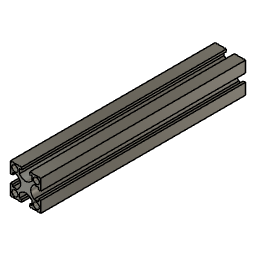
프로파일-135mm (Autodesk Fusion 360 design; units mm, degrees)
Autodesk Fusion 360 part; units mm, degrees
sketch "스케치1" plane through (0, 0, 0) normal (0, 1, 0) x (1, 0, 0)
  line L0 (10, -10) -> (-10, -10)
  line L1 (-10, -10) -> (-10, 10)
  line L2 (-10, 10) -> (10, 10)
  line L3 (10, 10) -> (10, -10)
  line L4 (10, -10) -> (-10, 10) construction
  line L5 (-10, -10) -> (10, 10) construction
  line L6 (10, 0) -> (10, -4.15)
  line L7 (3.3, 0) -> (3.3, 4.15)
  line L8 (3.3, 4.15) -> (10, 4.15)
  line L9 (10, 4.15) -> (10, -4.15)
  line L10 (10, -4.15) -> (3.3, -4.15)
  line L11 (3.3, -4.15) -> (3.3, 4.15)
  line L12 (10, -4.15) -> (8.5, -4.15)
  line L13 (8.5, -4.15) -> (8.5, -2.65)
  line L14 (8.5, -2.65) -> (10, -2.65)
  line L15 (10, -2.65) -> (10, -4.15)
  line L16 (10, 4.15) -> (8.5, 4.15)
  line L17 (8.5, 4.15) -> (8.5, 2.65)
  line L18 (8.5, 2.65) -> (10, 2.65)
  line L19 (10, 2.65) -> (10, 4.15)
  line L20 (8.5, 4.15) -> (5.5, 4.15)
  line L21 (5.5, 4.15) -> (5.5, -4.15)
  line L22 (5.5, -4.15) -> (8.5, -4.15)
  line L23 (8.5, -4.15) -> (8.5, 4.15)
  spline S0 degree 5 poles (5.5, -4.15) (5.3331, -3.984) (5.014, -3.652) (4.579, -3.154) (4.0878, -2.49) (3.6321, -1.66) (3.3486, -0.83) (3.2516, 0) (3.3486, 0.83) (3.6321, 1.66) (4.0878, 2.49) (4.579, 3.154) (5.014, 3.652) (5.3331, 3.984) (5.5, 4.15) knots 0 0 0 0 0 0 0.1 0.2 0.3 0.4 0.5 0.6 0.7 0.8 0.9 1 1 1 1 1 1
  spline S1 degree 5 poles (4.15, 5.5) (3.984, 5.3331) (3.652, 5.014) (3.154, 4.579) (2.49, 4.0878) (1.66, 3.6321) (0.83, 3.3486) (0, 3.2516) (-0.83, 3.3486) (-1.66, 3.6321) (-2.49, 4.0878) (-3.154, 4.579) (-3.652, 5.014) (-3.984, 5.3331) (-4.15, 5.5) knots 0 0 0 0 0 0 0.1 0.2 0.3 0.4 0.5 0.6 0.7 0.8 0.9 1 1 1 1 1 1
  line L24 (4.15, 5.5) -> (4.15, 8.5)
  line L25 (4.15, 8.5) -> (2.65, 8.5)
  line L26 (2.65, 8.5) -> (2.65, 10)
  line L27 (-4.15, 8.5) -> (-4.15, 5.5)
  line L28 (-4.15, 8.5) -> (-2.65, 8.5)
  line L29 (-2.65, 8.5) -> (-2.65, 10)
  spline S2 degree 5 poles (-5.5, 4.15) (-5.3331, 3.984) (-5.014, 3.652) (-4.579, 3.154) (-4.0878, 2.49) (-3.6321, 1.66) (-3.3486, 0.83) (-3.2516, 0) (-3.3486, -0.83) (-3.6321, -1.66) (-4.0878, -2.49) (-4.579, -3.154) (-5.014, -3.652) (-5.3331, -3.984) (-5.5, -4.15) knots 0 0 0 0 0 0 0.1 0.2 0.3 0.4 0.5 0.6 0.7 0.8 0.9 1 1 1 1 1 1
  line L30 (-5.5, 4.15) -> (-8.5, 4.15)
  line L31 (-8.5, 4.15) -> (-8.5, 2.65)
  line L32 (-8.5, 2.65) -> (-10, 2.65)
  line L33 (-8.5, -4.15) -> (-5.5, -4.15)
  line L34 (-8.5, -4.15) -> (-8.5, -2.65)
  line L35 (-8.5, -2.65) -> (-10, -2.65)
  spline S3 degree 5 poles (-4.15, -5.5) (-3.984, -5.3331) (-3.652, -5.014) (-3.154, -4.579) (-2.49, -4.0878) (-1.66, -3.6321) (-0.83, -3.3486) (0, -3.2516) (0.83, -3.3486) (1.66, -3.6321) (2.49, -4.0878) (3.154, -4.579) (3.652, -5.014) (3.984, -5.3331) (4.15, -5.5) knots 0 0 0 0 0 0 0.1 0.2 0.3 0.4 0.5 0.6 0.7 0.8 0.9 1 1 1 1 1 1
  line L36 (-4.15, -5.5) -> (-4.15, -8.5)
  line L37 (-4.15, -8.5) -> (-2.65, -8.5)
  line L38 (-2.65, -8.5) -> (-2.65, -10)
  line L39 (4.15, -8.5) -> (4.15, -5.5)
  line L40 (4.15, -8.5) -> (2.65, -8.5)
  line L41 (2.65, -8.5) -> (2.65, -10)
  line L42 (-10, -10) -> (-4.15, -10)
  line L43 (-4.15, -10) -> (-4.15, -4.15)
  line L44 (-4.15, -4.15) -> (-10, -4.15)
  line L45 (-10, -4.15) -> (-10, -10)
  circle A0 centre (-7.075, -7.075) radius 2
  circle A1 centre (7.075, -7.075) radius 2
  circle A2 centre (7.075, 7.075) radius 2
  circle A3 centre (-7.075, 7.075) radius 2
  point P0 (0, 3.3)
  point P1 (-3.3, 0)
  point P2 (0, -3.3)
  dimension "d1" = 20
  dimension "d2" = 20
  dimension "d3" = 6.7
  dimension "d4" = 4.15
  dimension "d5" = 4.15
  dimension "d6" = 1.5
  dimension "d7" = 1.5
  dimension "d8" = 1.5
  dimension "d9" = 1.5
  dimension "d10" = 3
  dimension "d12" = 360
  dimension "d13" = 5.85
  dimension "d14" = 4
  dimension "d16" = 360
  constraint horizontal L0
  constraint perpendicular L0 L1
  constraint parallel L0 L2
  constraint parallel L1 L3
  constraint coincident L4 origin
  constraint coincident L5 origin
  constraint midpoint L3 L6.start
  constraint horizontal L8
  constraint vertical L9
  constraint horizontal L10
  constraint vertical L11
  constraint horizontal L12
  constraint vertical L13
  constraint horizontal L14
  constraint vertical L15
  constraint horizontal L16
  constraint vertical L17
  constraint horizontal L18
  constraint vertical L19
  constraint horizontal L20
  constraint vertical L21
  constraint horizontal L22
  constraint vertical L23
  constraint horizontal L42
  constraint vertical L43
  constraint horizontal L44
  constraint vertical L45
  constraint coincident L5 A0.centre
  measures "d1" distance of L1.end L2.end
  measures "d2" distance of L0.end L1.end
  measures "d3" distance of L6.start L7.start
  measures "d4" distance of L6.start L6.end
  measures "d5" distance of L7.start L7.end
  measures "d6" distance of L6.end L12.end
  measures "d7" distance of L6.end L14.end
  measures "d8" distance of L8.end L16.end
  measures "d9" distance of L8.end L18.end
  measures "d10" distance of L16.end L20.end
  measures "d13" distance of L0.end L44.end
  measures "d14" diameter of A0
extrude "돌출1" add sketch "스케치1" along normal blind 135 contours L0 L1 L2 L3 L7 L8 L10 L11 L12 L16 L20 L22 S1 L24 L25 L26 L27 L28 L29 S2 L30 L31 L32 S3 L39 L40 L41 L43 L44 | L3 L6 L9 L10 L12 L13 L14 L15 L23 | L0 L37 L38 L43 | L0 L1 L33 L36 L42 L43 L44 L45 | L10 L11 S0 | L3 L8 L9 L16 L17 L18 L19 L23 | L7 L8 L11 S0 | L1 L34 L35 L44
